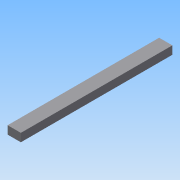
# Autodesk Inventor part: tigemoteur
Saved by Autodesk Inventor 2013 (Build 170138000, 138)
## iProperties
Created: 2012-11-14
Part Number: tigemoteur
Material: Générique
Document SubType Name: Modeling
Designer: Aegir
Density: 1 g/cm^3
Author: Aegir
Autodesk Inventor part; units mm, degrees
ref_plane "YZ Plane" through (0, 0, 0) normal (1, 0, 0) x (0, 1, 0)
ref_plane "XZ Plane" through (0, 0, 0) normal (0, 1, 0) x (-1, 0, 0)
ref_plane "XY Plane" through (0, 0, 0) normal (0, 0, 1) x (1, 0, 0)
sketch "Esquisse1" plane through (0, 0, 0) normal (0, 0, 1) x (1, 0, 0)
  line L0 (2.4067, 0) -> (-2.468, 0)
  line L1 (-2.468, 0) -> (-2.468, 55.8233)
  line L2 (-2.468, 55.8233) -> (2.4067, 55.8233)
  line L3 (2.4067, 55.8233) -> (2.4067, 0)
  point P0 (0, 0)
  constraints: 8 end point, 2 parallel, 1 horizontal, 1 perpendicular
extrude "Extrusion1" add sketch "Esquisse1" along normal blind 3
